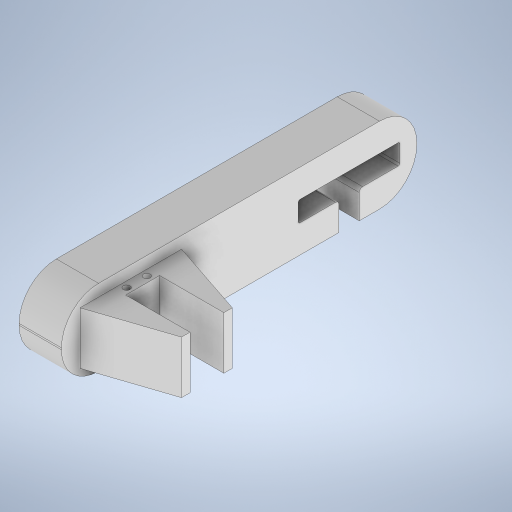
# Autodesk Inventor part: base
Saved by Autodesk Inventor 2023 (Build 270158000, 158)
## iProperties
Created: 2024-05-17
Part Number: base
Material: 一般
Document SubType Name: Modeling
Designer: cadlab
Density: 1 g/cm^3
Appearance: 預設
Author: cadlab
Autodesk Inventor part; units mm, degrees
ref_plane "YZ Plane" through (0, 0, 0) normal (1, 0, 0) x (0, 1, 0)
ref_plane "XZ Plane" through (0, 0, 0) normal (0, 1, 0) x (-1, 0, 0)
ref_plane "XY Plane" through (0, 0, 0) normal (0, 0, 1) x (1, 0, 0)
sketch "草圖1" plane through (0, 0, 0) normal (1, 0, 0) x (0, 1, 0)
  line L0 (-22.5, -105) -> (22.5, -105)
  line L1 (22.5, -105) -> (22.5, 105)
  line L2 (22.5, 105) -> (-22.5, 105)
  line L3 (-22.5, 105) -> (-22.5, -105)
  line L4 (-22.5, -105) -> (22.5, 105) construction
  line L5 (22.5, -105) -> (-22.5, 105) construction
  point P0 (0, 0)
  dimension "d0" = 210
  dimension "d1" = 45
  constraints: 12 end point, 2 midpoint, 2 parallel, 1 horizontal, 1 perpendicular
  measures "d0" distance of L0.end L1.end
  measures "d1" distance of L1.end L2.end
extrude "擠出1" add sketch "草圖1" along normal blind 25
fillet "圓角1" radius 22 4 edges at (12.5, 22.5, 105) (12.5, -22.5, 105) (12.5, 22.5, -105) (12.5, -22.5, -105)
sketch "草圖2" plane through (25, 0, 0) normal (1, 0, 0) x (0, 0, -1)
  line L0 (35, 6) -> (95, 6)
  line L1 (95, 6) -> (95, -6)
  line L2 (35, -6) -> (35, 6)
  line L3 (71, -6) -> (71, -22.5)
  line L4 (71, -22.5) -> (59, -22.5)
  line L5 (59, -22.5) -> (59, -6)
  line L6 (0, 0) -> (51.0559, 0) construction
  line L7 (95, -6) -> (71, -6)
  line L8 (59, -6) -> (35, -6)
  line L9 (65, -22.5) -> (65, 6) construction
  line L10 (-83, -22.5) -> (83, -22.5) construction
  line L11 (105, -0.5) -> (105, 0.5) projected
  dimension "d5" = 12
  dimension "d6" = 60
  dimension "d7" = 12
  dimension "d8" = 10
  constraints: 20 end point, 4 parallel, 3 horizontal, 2 collinear, 2 midpoint, 2 perpendicular, 1 vertical, 1 other
  measures "d5" distance of L0.end L1.end
  measures "d6" distance of L0.start L0.end
  measures "d7" distance of L3.end L4.end
  measures "d8" distance between parallel lines of L1 L11
extrude "擠出2" cut sketch "草圖2" against normal blind 25
fillet "圓角2" radius 1 4 edges at (12.5, 6, -35) (12.5, -6, -35) (12.5, 6, -95) (12.5, -6, -95)
fillet "圓角3" radius 2 2 edges at (12.5, -6, -59) (12.5, -6, -71)
sketch "草圖3" plane through (0, 0, 0) normal (0, 1, 0) x (-1, 0, 0)
  line L0 (-25, 94) -> (-25, 34)
  line L1 (-70, 79) -> (-25, 94)
  line L2 (-70, 49) -> (-25, 34)
  line L3 (-32, 74) -> (-70, 74)
  line L4 (-70, 54) -> (-32, 54)
  line L5 (-32, 54) -> (-32, 74)
  line L6 (-70, 49) -> (-70, 54)
  line L7 (-70, 74) -> (-70, 79)
  line L8 (-32, 64) -> (-25, 64) construction
  line L9 (-25, 83) -> (-25, -59) construction
  line L10 (0, -59) -> (-25, -59) projected
  point P0 (0, 0)
  dimension "d13" = 113
  dimension "d14" = 20
  dimension "d15" = 5
  dimension "d16" = 20
  dimension "d17" = 45
  dimension "d21" = 38
  constraints: 18 end point, 3 collinear, 3 parallel, 2 horizontal, 2 midpoint, 1 vertical
  measures "d13" distance from line of L10 L4.start
  measures "d14" vertical distance of L0.end L4.start
  measures "d15" distance of L2.start L4.start
  measures "d16" distance between parallel lines of L4 L3
  measures "d17" distance between parallel lines of L0 L7
  measures "d21" distance of L3.start L3.end
extrude "擠出3" add sketch "草圖3" along normal mid plane 31
sketch "草圖4" plane through (0, -15.5, 0) normal (0, -1, 0) x (1, 0, 0)
  circle A0 centre (28.5, 69.95) radius 2
  circle A1 centre (28.5, 58.05) radius 2
  line L0 (25, 105) -> (25, 83) construction
  line L1 (70, 64) -> (28.5, 64) construction
  line L2 (70, 74) -> (32, 74) construction
  line L3 (32, 54) -> (70, 54) construction
  point P0 (0, 0)
  dimension "d22" = 3.5
  dimension "d23" = 4
  dimension "d24" = 11.9
  dimension "d25" = 10
  constraints: 2 centre point, 2 end point, 2 vertical alignment, 1 equal radius, 1 horizontal, 1 other
  measures "d22" distance from line of A0.centre L0
  measures "d23" diameter of A0
  measures "d24" distance of A1.centre A0.centre
  measures "d25" distance between parallel lines of L1 L3
extrude "擠出4" cut sketch "草圖4" against normal blind 31
